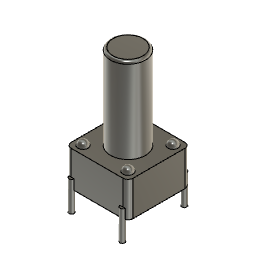
tactile_6x6x12 (Autodesk Fusion 360 design; units mm, degrees)
Autodesk Fusion 360 part; units mm, degrees
note: some values were not read from the file. Set by a fixed rule: which sketch regions a step uses.
sketch "スケッチ1" plane through (0, 0, 0) normal (0, 0, 1) x (1, 0, 0)
  line L0 (0, 0) -> (6.2, 0)
  line L1 (6.2, 0) -> (6.2, 6.2)
  line L2 (6.2, 6.2) -> (0, 6.2)
  line L3 (0, 6.2) -> (0, 0)
  circle A0 centre (0.56, 0) radius 0.25
  circle A1 centre (5.64, 0) radius 0.25
  line L4 (0.56, 0) -> (5.64, 0) construction
  line L5 (-0.8303, 3.1) -> (7.1697, 3.1) construction
  circle A2 centre (0.56, 6.2) radius 0.25
  circle A3 centre (5.64, 6.2) radius 0.25
  dimension "d1" = 6.2
  dimension "d2" = 6.2
  dimension "d10" = 0.5
  dimension "d11" = 5.08
  dimension "d12" = 0.56
  dimension "d13" = 3.1
  constraint horizontal L0
  constraint vertical L1
  constraint horizontal L2
  constraint vertical L3
  constraint coincident L0.start L3.end
  constraint equal A0 A1
  constraint coincident L0 A0.centre
  constraint coincident L0 A1.centre
  constraint coincident A0.centre L4.start
  constraint coincident A1.centre L4.end
  constraint perpendicular L1 L5
  constraint symmetric A0 L5 A2
  constraint symmetric A1 L5 A3
  measures "d1" distance of L0.start L0.end
  measures "d2" distance of L0.start L2.end
  measures "d10" diameter of A0
  measures "d11" distance of A0.centre A1.centre
  measures "d12" distance of L0.start A0.centre
  measures "d13" distance of L2 L5
extrude "押し出し1" add sketch "スケッチ1" along normal blind 3.5 contours L0 L1 L2 L3 A0 A1 A2 A3 | L0 A1 | L0 A0 | L2 A3 | L2 A2 picked at (5.7011, 0.0567) picked at (0.6211, 0.0567) picked at (5.588, 6.0857) picked at (0.5126, 6.0741)
sketch "スケッチ2" plane through (0, 0, 3.5) normal (0, 0, 1) x (-1, 0, 0)
  line L0 (0, -6.2) -> (0, 0)
  line L1 (0, 0) -> (-6.2, 0)
  line L2 (-6.2, 0) -> (-6.2, -6.2)
  line L3 (-6.2, -6.2) -> (0, -6.2)
  circle A0 centre (-3.1, -3.1) radius 1.75
  circle A1 centre (-0.85, -5.35) radius 0.5
  circle A2 centre (-5.35, -5.35) radius 0.5
  circle A3 centre (-5.35, -0.85) radius 0.5
  circle A4 centre (-0.85, -0.85) radius 0.5
  line L4 (0, -6.2) -> (0, 0)
  line L5 (-6.9311, -0.85) -> (1.5036, -0.85) construction
  line L6 (-0.56, 0) -> (-5.64, 0)
  line L7 (-0.85, -6.8597) -> (-0.85, 0.6131) construction
  dimension "d5" = 3.5
  dimension "d6" = 3.1
  dimension "d7" = 3.1
  dimension "d19" = 1
  dimension "d20" = 4.5
  dimension "d22" = 0.85
  dimension "d23" = 0.85
  dimension "d24" = 4.5
  dimension "d25" = 4.5
  dimension "d26" = 4.5
  constraint equal A3 A4
  constraint equal A2 A4
  constraint equal A1 A4
  constraint horizontal L5
  constraint coincident A4.centre L5
  constraint vertical L7
  constraint coincident A4.centre L7
  constraint coincident A1.centre L7
  constraint coincident A3.centre L5
  measures "d5" diameter of A0
  measures "d6" distance of L1 A0.centre
  measures "d7" distance of L0 A0.centre
  measures "d19" diameter of A4
  measures "d20" distance of A3.centre A4.centre
  measures "d22" distance of L5 L6
  measures "d23" distance of L4 L7
  measures "d24" vertical distance of A2.centre A3.centre
  measures "d25" distance of A1.centre A4.centre
  measures "d26" distance of A1.centre A2.centre
extrude "押し出し2" add sketch "スケッチ2" along normal blind 8.5 contours A0
extrude "押し出し3" add sketch "スケッチ1" against normal blind 2 contours L0 A1 | L0 A1 | L0 A0 | L0 A0 | L2 A3 | L2 A3 | L2 A2 | L2 A2
extrude "押し出し4" add sketch "スケッチ1" along normal blind 1 contours L0 A1 | L0 A0 | L2 A3 | L2 A2 picked at (5.588, -0.0652) picked at (0.4911, -0.0469) picked at (5.7011, 6.3058) picked at (0.636, 6.2486)
extrude "押し出し5" add sketch "スケッチ2" along normal blind 0.5 contours A1 | A2 | A3 | A4
fillet "フィレット1" radius 0.5 4 edges at (5.8162, 1.0308, 4) (1.3162, 1.0308, 4) (1.3162, 5.5308, 4) (5.8162, 5.5308, 4)
fillet "フィレット2" radius 0.5 4 edges at (6.2, 0, 1.75) (6.2, 6.2, 1.75) (0, 0, 1.75) (0, 6.2, 1.75)
fillet "フィレット3" radius 0.25 1 edges at (4.7316, 3.7328, 12)
